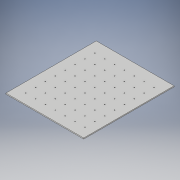
# Autodesk Inventor part: Drawer
Saved by Autodesk Inventor 2018 (Build 220112000, 112)
## iProperties
Created: 2018-04-30
Part Number: Drawer
Material: Generic
Document SubType Name: Modeling
Designer: bbramman
Density: 1 g/cm^3
Appearance: Default
Author: bbramman
Autodesk Inventor part; units mm, degrees
ref_plane "YZ Plane" through (0, 0, 0) normal (1, 0, 0) x (0, 1, 0)
ref_plane "XZ Plane" through (0, 0, 0) normal (0, 1, 0) x (-1, 0, 0)
ref_plane "XY Plane" through (0, 0, 0) normal (0, 0, 1) x (1, 0, 0)
sketch "Sketch1" plane through (0, 0, 0) normal (0, 1, 0) x (-1, 0, 0)
  line L0 (-200, 232.41) -> (200, 232.41)
  line L1 (200, 232.41) -> (200, -232.41)
  line L2 (200, -232.41) -> (-200, -232.41)
  line L3 (-200, -232.41) -> (-200, 232.41)
  line L4 (-200, 232.41) -> (200, -232.41) construction
  line L5 (200, 232.41) -> (-200, -232.41) construction
  point P0 (0, 0)
  dimension "d0" = 400
  dimension "d1" = 464.82
  constraints: 12 end point, 2 midpoint, 2 parallel, 1 horizontal, 1 perpendicular
  measures "d0" distance of L1.end L2.end
  measures "d1" distance of L0.end L1.end
extrude "Extrusion1" add sketch "Sketch1" along normal blind 5.08
sketch "Sketch2" plane through (0, 5.08, 0) normal (0, 1, 0) x (1, 0, 0)
  circle A0 centre (-149.1996, -181.61) radius 2.0828
  circle A1 centre (-149.1996, -130.81) radius 2.0828
  circle A2 centre (-149.1996, -80.01) radius 2.0828
  circle A3 centre (-149.1996, -29.21) radius 2.0828
  circle A4 centre (-149.1996, 21.59) radius 2.0828
  circle A5 centre (-149.1996, 72.39) radius 2.0828
  circle A6 centre (-149.1996, 123.19) radius 2.0828
  circle A7 centre (-149.1996, 173.99) radius 2.0828
  circle A8 centre (-98.3996, -181.61) radius 2.0828
  circle A9 centre (-98.3996, -130.81) radius 2.0828
  circle A10 centre (-98.3996, -80.01) radius 2.0828
  circle A11 centre (-98.3996, -29.21) radius 2.0828
  circle A12 centre (-98.3996, 21.59) radius 2.0828
  circle A13 centre (-98.3996, 72.39) radius 2.0828
  circle A14 centre (-98.3996, 123.19) radius 2.0828
  circle A15 centre (-98.3996, 173.99) radius 2.0828
  circle A16 centre (-47.5996, -181.61) radius 2.0828
  circle A17 centre (-47.5996, -130.81) radius 2.0828
  circle A18 centre (-47.5996, -80.01) radius 2.0828
  circle A19 centre (-47.5996, -29.21) radius 2.0828
  circle A20 centre (-47.5996, 21.59) radius 2.0828
  circle A21 centre (-47.5996, 72.39) radius 2.0828
  circle A22 centre (-47.5996, 123.19) radius 2.0828
  circle A23 centre (-47.5996, 173.99) radius 2.0828
  circle A24 centre (3.2004, 173.99) radius 2.0828
  circle A25 centre (3.2004, 123.19) radius 2.0828
  circle A26 centre (3.2004, 72.39) radius 2.0828
  circle A27 centre (3.2004, 21.59) radius 2.0828
  circle A28 centre (3.2004, -29.21) radius 2.0828
  circle A29 centre (3.2004, -80.01) radius 2.0828
  circle A30 centre (3.2004, -130.81) radius 2.0828
  circle A31 centre (3.2004, -181.61) radius 2.0828
  circle A32 centre (54.0004, -181.61) radius 2.0828
  circle A33 centre (54.0004, -130.81) radius 2.0828
  circle A34 centre (54.0004, -80.01) radius 2.0828
  circle A35 centre (54.0004, -29.21) radius 2.0828
  circle A36 centre (54.0004, 21.59) radius 2.0828
  circle A37 centre (54.0004, 72.39) radius 2.0828
  circle A38 centre (54.0004, 123.19) radius 2.0828
  circle A39 centre (54.0004, 173.99) radius 2.0828
  circle A40 centre (104.8004, 173.99) radius 2.0828
  circle A41 centre (104.8004, 123.19) radius 2.0828
  circle A42 centre (104.8004, 72.39) radius 2.0828
  circle A43 centre (104.8004, 21.59) radius 2.0828
  circle A44 centre (104.8004, -29.21) radius 2.0828
  circle A45 centre (104.8004, -80.01) radius 2.0828
  circle A46 centre (104.8004, -130.81) radius 2.0828
  circle A47 centre (104.8004, -181.61) radius 2.0828
  circle A48 centre (155.6004, -181.61) radius 2.0828
  circle A49 centre (155.6004, -130.81) radius 2.0828
  circle A50 centre (155.6004, -80.01) radius 2.0828
  circle A51 centre (155.6004, -29.21) radius 2.0828
  circle A52 centre (155.6004, 21.59) radius 2.0828
  circle A53 centre (155.6004, 72.39) radius 2.0828
  circle A54 centre (155.6004, 123.19) radius 2.0828
  circle A55 centre (155.6004, 173.99) radius 2.0828
  point P0 (0, 0)
  dimension "d4" = 4.1656
  dimension "d5" = 4.1656
  dimension "d6" = 4.1656
  dimension "d7" = 4.1656
  dimension "d8" = 4.1656
  dimension "d9" = 4.1656
  dimension "d10" = 4.1656
  dimension "d11" = 4.1656
  dimension "d12" = 4.1656
  dimension "d13" = 4.1656
  dimension "d14" = 4.1656
  dimension "d15" = 4.1656
  dimension "d16" = 4.1656
  dimension "d17" = 4.1656
  dimension "d18" = 4.1656
  dimension "d19" = 4.1656
  dimension "d20" = 4.1656
  dimension "d21" = 4.1656
  dimension "d22" = 4.1656
  dimension "d23" = 4.1656
  dimension "d24" = 4.1656
  dimension "d25" = 4.1656
  dimension "d26" = 4.1656
  dimension "d27" = 4.1656
  dimension "d28" = 4.1656
  dimension "d29" = 4.1656
  dimension "d30" = 4.1656
  dimension "d31" = 4.1656
  dimension "d32" = 4.1656
  dimension "d33" = 4.1656
  dimension "d34" = 4.1656
  dimension "d35" = 4.1656
  dimension "d36" = 4.1656
  dimension "d37" = 4.1656
  dimension "d38" = 4.1656
  dimension "d39" = 4.1656
  dimension "d40" = 4.1656
  dimension "d41" = 4.1656
  dimension "d42" = 4.1656
  dimension "d43" = 4.1656
  dimension "d44" = 4.1656
  dimension "d45" = 4.1656
  dimension "d46" = 4.1656
  dimension "d47" = 4.1656
  dimension "d48" = 4.1656
  dimension "d49" = 4.1656
  dimension "d50" = 4.1656
  dimension "d51" = 4.1656
  dimension "d52" = 4.1656
  dimension "d53" = 4.1656
  dimension "d54" = 4.1656
  dimension "d55" = 4.1656
  dimension "d56" = 4.1656
  dimension "d57" = 4.1656
  dimension "d58" = 4.1656
  dimension "d59" = 4.1656
  constraints: 56 centre point, 56 coincident
  measures "d4" diameter of A0
  measures "d5" diameter of A1
  measures "d6" diameter of A2
  measures "d7" diameter of A3
  measures "d8" diameter of A4
  measures "d9" diameter of A5
  measures "d10" diameter of A6
  measures "d11" diameter of A7
  measures "d12" diameter of A8
  measures "d13" diameter of A9
  measures "d14" diameter of A10
  measures "d15" diameter of A11
  measures "d16" diameter of A12
  measures "d17" diameter of A13
  measures "d18" diameter of A14
  measures "d19" diameter of A15
  measures "d20" diameter of A16
  measures "d21" diameter of A17
  measures "d22" diameter of A18
  measures "d23" diameter of A19
  measures "d24" diameter of A20
  measures "d25" diameter of A21
  measures "d26" diameter of A22
  measures "d27" diameter of A23
  measures "d28" diameter of A24
  measures "d29" diameter of A25
  measures "d30" diameter of A26
  measures "d31" diameter of A27
  measures "d32" diameter of A28
  measures "d33" diameter of A29
  measures "d34" diameter of A30
  measures "d35" diameter of A31
  measures "d36" diameter of A32
  measures "d37" diameter of A33
  measures "d38" diameter of A34
  measures "d39" diameter of A35
  measures "d40" diameter of A36
  measures "d41" diameter of A37
  measures "d42" diameter of A38
  measures "d43" diameter of A39
  measures "d44" diameter of A40
  measures "d45" diameter of A41
  measures "d46" diameter of A42
  measures "d47" diameter of A43
  measures "d48" diameter of A44
  measures "d49" diameter of A45
  measures "d50" diameter of A46
  measures "d51" diameter of A47
  measures "d52" diameter of A48
  measures "d53" diameter of A49
  measures "d54" diameter of A50
  measures "d55" diameter of A51
  measures "d56" diameter of A52
  measures "d57" diameter of A53
  measures "d58" diameter of A54
  measures "d59" diameter of A55
extrude "Extrusion2" cut sketch "Sketch2" against normal through all
body "Solid1"
